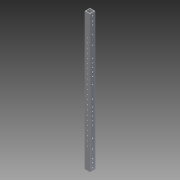
# Autodesk Inventor part: Chassis Part1 (26x28)
Saved by Autodesk Inventor 2013 (Build 170138000, 138)
## iProperties
Created: 2013-01-05
Part Number: Chassis Part1 (26x28)
Material: Aluminum 6061
Document SubType Name: Modeling
Designer: Moses
Density: 2.71 g/cm^3
Mass: 452.147 g
Surface Area: 1088.25 cm^2
Volume: 166.844 cm^3
Author: Moses
Autodesk Inventor part; units mm, degrees
ref_plane "YZ Plane" through (0, 0, 0) normal (1, 0, 0) x (0, 1, 0)
ref_plane "XZ Plane" through (0, 0, 0) normal (0, 1, 0) x (-1, 0, 0)
ref_plane "XY Plane" through (0, 0, 0) normal (0, 0, 1) x (1, 0, 0)
sketch "Sketch1" plane through (0, 0, 0) normal (0, 1, 0) x (-1, 0, 0)
  line L0 (0, 25.4) -> (25.4, 25.4)
  line L1 (25.4, 25.4) -> (25.4, 0)
  line L2 (25.4, 0) -> (0, 0)
  line L3 (0, 0) -> (0, 25.4)
  line L4 (22.225, 22.225) -> (3.175, 22.225)
  line L5 (3.175, 22.225) -> (3.175, 3.175)
  line L6 (3.175, 3.175) -> (22.225, 3.175)
  line L7 (22.225, 3.175) -> (22.225, 22.225)
  dimension "d0" = 25.4
  dimension "d1" = 25.4
  dimension "d2" = 3.175
  constraints: 16 end point, 4 parallel, 2 perpendicular, 1 coincident, 1 horizontal, 3 other
  measures "d0" distance of L1.end L2.end
  measures "d1" distance of L0.end L1.end
  measures "d2" distance between parallel lines of L0 L4
extrude "Extrusion1" add sketch "Sketch1" along normal blind 660.4
sketch "Sketch2" plane through (-25.4, 0, 25.4) normal (0, 0, 1) x (1, 0, 0)
  circle A0 centre (12.7, 534.8581) radius 3.302 projected
  circle A1 centre (12.7, 491.7722) radius 3.302 projected
  circle A2 centre (12.7, 448.6863) radius 3.302 projected
  circle A3 centre (12.7, 405.6004) radius 3.302 projected
  circle A4 centre (12.7, 362.5144) radius 3.302 projected
  circle A5 centre (12.7, 319.4285) radius 3.302 projected
  circle A6 centre (12.7, 276.3426) radius 3.302 projected
  circle A7 centre (12.7, 233.2567) radius 3.302 projected
  circle A8 centre (12.7, 190.1707) radius 3.302 projected
  circle A9 centre (12.7, 147.0848) radius 3.302 projected
  circle A10 centre (12.7, 103.9989) radius 3.302 projected
  circle A11 centre (12.7, 125.5419) radius 3.302 projected
  circle A12 centre (12.7, 168.6278) radius 3.302 projected
  circle A13 centre (12.7, 211.7137) radius 3.302 projected
  circle A14 centre (12.7, 254.7996) radius 3.302 projected
  circle A15 centre (12.7, 297.8856) radius 3.302 projected
  circle A16 centre (12.7, 340.9715) radius 3.302 projected
  circle A17 centre (12.7, 384.0574) radius 3.302 projected
  circle A18 centre (12.7, 427.1433) radius 3.302 projected
  circle A19 centre (12.7, 470.2293) radius 3.302 projected
  circle A20 centre (12.7, 513.3152) radius 3.302 projected
  circle A21 centre (12.7, 556.4011) radius 3.302 projected
  line L0 (25.4, 25.4) -> (0, 25.4) projected
  line L1 (25.4, 25.4) -> (25.4, 635) projected
  line L2 (0, 635) -> (25.4, 635) projected
  line L3 (0, 25.4) -> (0, 635) projected
extrude "Extrusion2" cut sketch "Sketch2" against normal through all contours A0 | A1 | A2 | A3 | A4 | A5 | A6 | A7 | A8 | A9 | A10 | A11 | A12 | A13 | A14 | A15 | A16 | A17 | A18 | A19 | A20 | A21
sketch "Sketch3" plane through (-25.4, 0, 0) normal (-1, 0, 0) x (0, 0, 1)
  line L0 (25.4, 0) -> (25.4, 660.4) projected
  line L1 (0, 0) -> (0, 660.4) projected
  line L2 (0, 556.4011) -> (25.4, 556.4011) construction
  line L3 (0, 405.6004) -> (25.4, 405.6004) construction
  line L4 (0, 254.7996) -> (25.4, 254.7996) construction
  line L5 (0, 103.9989) -> (25.4, 103.9989) construction
  line L6 (12.7, 569.1011) -> (12.7, 524.6511) construction
  line L7 (12.7, 435.7629) -> (12.7, 375.4379) construction
  line L8 (12.7, 277.0246) -> (12.7, 232.5746) construction
  line L9 (12.7, 135.7489) -> (12.7, 91.2989) construction
  circle A0 centre (12.7, 569.1011) radius 3.302
  circle A1 centre (12.7, 524.6511) radius 3.302
  circle A2 centre (12.7, 435.7629) radius 3.302
  circle A3 centre (12.7, 375.4379) radius 3.302
  circle A4 centre (12.7, 277.0246) radius 3.302
  circle A5 centre (12.7, 232.5746) radius 3.302
  circle A6 centre (12.7, 135.7489) radius 3.302
  circle A7 centre (12.7, 91.2989) radius 3.302
  line L10 (0, 330.2) -> (25.4, 330.2) construction
  line L11 (12.7, 360.3625) -> (12.7, 300.0375) construction
  circle A8 centre (12.7, 360.3625) radius 3.302
  circle A9 centre (12.7, 300.0375) radius 3.302
  line L12 (0, 660.4) -> (25.4, 660.4) projected
  line L13 (0, 113.5239) -> (25.4, 113.5239) construction
  line L14 (25.4, 0) -> (0, 0) projected
  line L15 (0, 546.8761) -> (25.4, 546.8761) construction
  circle A10 centre (12.7, 12.7) radius 3.302 projected
  circle A11 centre (12.7, 34.925) radius 3.302 projected
  circle A12 centre (12.7, 50.8) radius 3.302 projected
  line L16 (22.225, 553.0991) -> (22.225, 559.7031) projected
  line L17 (22.225, 402.2984) -> (22.225, 408.9024) projected
  line L18 (22.225, 251.4976) -> (22.225, 258.1016) projected
  line L19 (22.225, 100.6969) -> (22.225, 107.3009) projected
  circle A13 centre (12.7, 647.7) radius 3.302 projected
  circle A14 centre (12.7, 625.475) radius 3.302 projected
  circle A15 centre (12.7, 609.6) radius 3.302 projected
  point P0 (12.7, 254.7996)
  point P1 (12.7, 405.6004)
  point P2 (12.7, 330.2)
  point P3 (12.7, 113.5239)
  point P4 (12.7, 546.8761)
  point P5 (22.225, 556.4011)
  point P6 (22.225, 405.6004)
  point P7 (22.225, 254.7996)
  point P8 (22.225, 103.9989)
  dimension "d7" = 44.45
  dimension "d8" = 60.325
  dimension "d9" = 44.45
  dimension "d10" = 44.45
  dimension "d11" = 6.604
  dimension "d12" = 6.604
  dimension "d13" = 6.604
  dimension "d14" = 6.604
  dimension "d15" = 6.604
  dimension "d16" = 6.604
  dimension "d17" = 6.604
  dimension "d18" = 6.604
  dimension "d21" = 60.325
  dimension "d22" = 6.604
  dimension "d23" = 6.604
  dimension "d27" = 9.525
  dimension "d28" = 9.525
  constraints: 24 end point, 14 midpoint, 10 centre point, 10 coincident, 4 point on line, 3 collinear, 3 horizontal, 3 parallel, 2 perpendicular, 16 other
  measures "d7" distance of L6.start L6.end
  measures "d8" distance of L7.start L7.end
  measures "d9" distance of L8.start L8.end
  measures "d10" distance of L9.start L9.end
  measures "d11" diameter of A0
  measures "d12" diameter of A1
  measures "d13" diameter of A2
  measures "d14" diameter of A3
  measures "d15" diameter of A4
  measures "d16" diameter of A5
  measures "d17" diameter of A6
  measures "d18" diameter of A7
  measures "d21" distance of L11.start L11.end
  measures "d22" diameter of A8
  measures "d23" diameter of A9
  measures "d27" distance between parallel lines of L5 L13
  measures "d28" distance between parallel lines of L15 L2
extrude "Extrusion3" cut sketch "Sketch3" against normal blind 25.4 contours A0 | A1 | A6 | A7 | A8 | A9 | A10 | A11 | A12 | A13 | A14 | A15
sketch "Sketch4" plane through (0, 0, 25.4) normal (1, 0, 0) x (0, 0, -1)
  line L0 (25.4, 0) -> (25.4, 660.4) projected
  line L1 (0, 0) -> (0, 660.4) projected
  line L2 (0, 330.2) -> (25.4, 330.2) construction
  line L3 (12.7, 374.65) -> (12.7, 285.75) construction
  circle A0 centre (12.7, 374.65) radius 3.302
  circle A1 centre (12.7, 285.75) radius 3.302
  circle A2 centre (12.7, 393.7) radius 3.302
  circle A3 centre (12.7, 412.75) radius 3.302
  circle A4 centre (12.7, 431.8) radius 3.302
  circle A5 centre (12.7, 450.85) radius 3.302
  circle A6 centre (12.7, 469.9) radius 3.302
  circle A7 centre (12.7, 266.7) radius 3.302
  circle A8 centre (12.7, 247.65) radius 3.302
  circle A9 centre (12.7, 228.6) radius 3.302
  circle A10 centre (12.7, 209.55) radius 3.302
  circle A11 centre (12.7, 190.5) radius 3.302
  point P0 (12.7, 330.2)
  dimension "d33" = 88.9
  dimension "d34" = 6.604
  dimension "d37" = 19.05
  dimension "d44" = 19.05
  constraints: 12 centre point, 4 end point, 4 midpoint, 2 coincident, 2 vertical, 1 equal radius, 1 perpendicular, 20 other
  measures "d33" distance of L3.start L3.end
  measures "d34" diameter of A0
  measures "d37" distance of A0.centre A2.centre
  measures "d44" distance of A1.centre A7.centre
extrude "Extrusion4" cut sketch "Sketch4" against normal blind 25.4 contours A2 | A3 | A4 | A5 | A6 | A7 | A8 | A9 | A10 | A11
equation "\"d9\" = d7"
equation "\"d10\" = d7"
equation "\"d12\" = d11"
equation "\"d13\" = d11"
equation "\"d14\" = d11"
equation "\"d15\" = d11"
equation "\"d16\" = d11"
equation "\"d17\" = d11"
equation "\"d18\" = d11"
equation "\"d21\" = d8"
equation "\"d22\" = d11"
equation "\"d23\" = d11"
equation "\"d27\" = d28"
body "Solid1"
